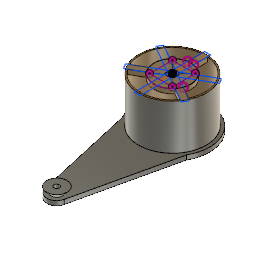
tulppajakiristinhuuli v2 (Autodesk Fusion 360 design; units mm, degrees)
Autodesk Fusion 360 part; units mm, degrees
note: some values were not read from the file. Set by a fixed rule: which sketch regions a step uses.
sketch "Sketch1" plane through (0, 0, 0) normal (0, 0, 1) x (1, 0, 0)
  circle A0 centre (0, 0) radius 48.5
  circle A1 centre (0, 0) radius 44.15
  circle A2 centre (0, 0) radius 42.15
  circle A3 centre (0, 0) radius 24
  line L0 (-4, 0) -> (4, 0)
  line L1 (4, 0) -> (4, 46)
  line L2 (4, 46) -> (-4, 46)
  line L3 (-4, 46) -> (-4, 0)
  line L4 (-2, 3.4641) -> (-41.8372, -19.5359)
  line L5 (-41.8372, -19.5359) -> (-37.8372, -26.4641)
  line L6 (-37.8372, -26.4641) -> (2, -3.4641)
  line L7 (2, -3.4641) -> (-2, 3.4641)
  line L8 (-2, -3.4641) -> (37.8372, -26.4641)
  line L9 (37.8372, -26.4641) -> (41.8372, -19.5359)
  line L10 (41.8372, -19.5359) -> (2, 3.4641)
  line L11 (2, 3.4641) -> (-2, -3.4641)
  circle A4 centre (0, 0) radius 6
  line L12 (15, 15) -> (-15, 15)
  line L13 (-15, 15) -> (-15, -15)
  line L14 (-15, -15) -> (15, -15)
  line L15 (15, -15) -> (15, 15)
  line L16 (15, 15) -> (-15, -15) construction
  line L17 (-15, 15) -> (15, -15) construction
  dimension "d1" = 97
  dimension "d2" = 88.3
  dimension "d3" = 84.3
  dimension "d4" = 48
  dimension "d6" = 360
  dimension "d7" = 12
  dimension "d12" = 30
  dimension "d13" = 30
  constraint coincident A0.centre A1.centre
  constraint concentric A1 A2
  constraint horizontal L0
  constraint vertical L1
  constraint horizontal L2
  constraint vertical L3
  constraint concentric A1 A4
  constraint perpendicular L12 L13
  constraint parallel L12 L14
  constraint parallel L13 L15
  constraint horizontal L12
  constraint coincident L16 A0.centre
  constraint coincident L17 A0.centre
  measures "d1" diameter of A0
  measures "d2" diameter of A1
  measures "d3" diameter of A2
  measures "d4" diameter of A3
  measures "d7" diameter of A4
  measures "d12" distance of L13.end L14.end
  measures "d13" distance of L12.end L13.end
extrude "Extrude1" add sketch "Sketch1" along normal blind 6 contours A0 | A1 L1 L2 L3 | A1 L8 L9 L10 | A2 A3 L1 L3 | A2 A3 L8 L10 | A1 L4 L5 L6 | A2 A3 L4 L6 | L1 L10 A4 L12 L15 | L1 L3 A4 L12 | L8 L10 A4 L15 | L3 L4 A4 L12 L13 | L6 L8 A4 L13 L14 L15 | L4 L6 A4 L13 makes body 1 at (48.4397, -2.4175, 4) makes body 2 at (-3.113, 29.8622, 0) makes body 3 at (-0.1495, -11.9944, 0) makes body 4 at (-27.4179, -12.2352, 0) makes body 5 at (27.4179, -12.2352, 0)
extrude "Extrude6" add sketch "Sketch1" along normal blind 6 contours A3 L1 L3 L12 | A3 L1 L10 L12 L15 | A3 L8 L10 L15 | A3 L3 L4 L12 L13 | A3 L6 L8 L13 L14 L15 | A3 L4 L6 L13 bodies 3 4 2 5
sketch "Sketch2" plane through (0, 0, 0) normal (0, 0, 1) x (1, 0, 0)
extrude "Extrude2" add sketch "Sketch1" along normal blind 65 contours A1 A2 L1 L10 | A1 A2 L1 L3 | A1 A2 L8 L10 | A1 A2 L3 L4 | A1 A2 L6 L8 | A1 A2 L4 L6 bodies 1 3
sketch "Sketch4" plane through (0, 0, 65) normal (0, 0, 1) x (-1, 0, 0)
  circle A0 centre (0, 0) radius 42.15
  circle A1 centre (0, 0) radius 44.15
  line L0 (-3.9193, -45.9529) -> (3.9193, -45.9529)
  line L1 (3.9193, -45.9529) -> (3.9193, 45.9529)
  line L2 (3.9193, 45.9529) -> (-3.9193, 45.9529)
  line L3 (-3.9193, 45.9529) -> (-3.9193, -45.9529)
  line L4 (-3.9193, -45.9529) -> (3.9193, 45.9529) construction
  line L5 (3.9193, -45.9529) -> (-3.9193, 45.9529) construction
  line L6 (41.7561, 19.5823) -> (37.8368, 26.3707)
  line L7 (-37.8368, -26.3707) -> (41.7561, 19.5823)
  line L8 (37.8368, 26.3707) -> (-41.7561, -19.5823)
  line L9 (-41.7561, -19.5823) -> (-37.8368, -26.3707)
  line L10 (-37.8368, 26.3707) -> (-41.7561, 19.5823)
  line L11 (41.7561, -19.5823) -> (-37.8368, 26.3707)
  line L12 (-41.7561, 19.5823) -> (37.8368, -26.3707)
  line L13 (37.8368, -26.3707) -> (41.7561, -19.5823)
  circle A2 centre (0, 0) radius 6
  circle A3 centre (0, 0) radius 24
  line L14 (-15, 15) -> (15, 15)
  line L15 (15, 15) -> (15, -15)
  line L16 (15, -15) -> (-15, -15)
  line L17 (-15, -15) -> (-15, 15)
  line L18 (-15, 15) -> (15, -15) construction
  line L19 (15, 15) -> (-15, -15) construction
  dimension "d20" = 360
  dimension "d21" = 12
  dimension "d22" = 48
  dimension "d25" = 30
  dimension "d26" = 30
  constraint perpendicular L0 L1
  constraint parallel L0 L2
  constraint parallel L1 L3
  constraint horizontal L0
  constraint coincident L4 A0.centre
  constraint coincident L5 A0.centre
  constraint coincident A0.centre A1.centre
  constraint concentric A0 A2
  constraint concentric A0 A3
  constraint perpendicular L14 L15
  constraint parallel L14 L16
  constraint parallel L15 L17
  constraint horizontal L14
  constraint coincident L18 A0.centre
  constraint coincident L19 A0.centre
  measures "d21" diameter of A2
  measures "d22" diameter of A3
  measures "d25" distance of L15.end L16.end
  measures "d26" distance of L14.end L15.end
extrude "Extrude4" add sketch "Sketch4" against normal blind 6 contours A0 L7 L8 A3 | L7 L11 A3 L15 | L7 L8 A3 L15 | L11 L12 A3 L15 | L1 L8 A3 L14 L15 | A0 L1 L3 A3 | L1 L12 A3 L15 L16 | L1 L3 A3 L14 | L1 L3 A3 L16 | A0 L11 L12 A3 | L3 L11 A3 L14 L17 | L3 L7 A3 L16 L17 | L11 L12 A3 L17 | L7 L8 A3 L17 | L8 L12 A3 L17 picked at (24.3429, 17.5763) picked at (3.0501, -29.8698) picked at (-27.393, 12.2934) bodies 1
sketch "Sketch5" plane through (0, 0, 65) normal (0, 0, 1) x (-1, 0, 0)
  arc A0 (3.9193, -41.9674) -> (38.3045, 17.5895) centre (0, 0) ccw
  line L0 (3.9193, -41.9674) -> (3.9193, -23.6778)
  arc A1 (3.9193, -23.6778) -> (22.4652, 8.4447) centre (0, 0) ccw
  line L1 (22.4652, 8.4447) -> (38.3045, 17.5895)
  line L2 (34.3852, 24.3779) -> (18.5459, 15.2331)
  line L3 (-18.5459, 15.2331) -> (-34.3852, 24.3779)
  arc A2 (34.3852, 24.3779) -> (-34.3852, 24.3779) centre (0, 0) ccw
  line L4 (-38.3045, 17.5895) -> (-22.4652, 8.4447)
  arc A3 (-22.4652, 8.4447) -> (-3.9193, -23.6778) centre (0, 0) ccw
  line L5 (-3.9193, -23.6778) -> (-3.9193, -41.9674)
  arc A4 (-38.3045, 17.5895) -> (-3.9193, -41.9674) centre (0, 0) ccw
  circle A5 centre (0, 0) radius 44.15
  arc A6 (18.5459, 15.2331) -> (-18.5459, 15.2331) centre (0, 0) ccw
  line L6 (15, -15) -> (-15, -15)
  line L7 (-15, -15) -> (-15, 15)
  line L8 (-15, 15) -> (15, 15)
  line L9 (15, 15) -> (15, -15)
extrude "Extrude5" add sketch "Sketch4" against normal blind 3 contours L7 L11 L15 | L1 L7 L8 L11 A2 L15 | L1 L7 L11 L12 A2 L15 | L1 L8 L14 L15 | L7 L11 A2 | L1 L12 L15 L16 | L1 L3 L8 L11 A2 L14 | L1 L8 A2 | L1 L3 L7 L12 A2 L16 | L1 L12 A2 | L3 L11 L14 L17 | L3 L7 L16 L17 | L3 L8 L11 L12 A2 L17 | L3 L11 A2 | L3 L7 L8 L12 A2 L17 | L3 L7 A2 | L8 L12 L17 | L8 L12 A2 bodies 1
extrude "Extrude7" add sketch "Sketch4" against normal blind 6 contours L7 L11 L15 | L1 L7 L8 L11 A2 L15 | L1 L7 L11 L12 A2 L15 | L1 L8 L14 L15 | L7 L11 A2 | L1 L12 L15 L16 | L1 L3 L8 L11 A2 L14 | L1 L8 A2 | L1 L3 L7 L12 A2 L16 | L1 L12 A2 | L3 L11 L14 L17 | L3 L7 L16 L17 | L3 L8 L11 L12 A2 L17 | L3 L11 A2 | L3 L7 L8 L12 A2 L17 | L3 L7 A2 | L8 L12 L17 | L8 L12 A2 bodies 1
sketch "Sketch8" plane through (0, 0, 0) normal (0, 0, 1) x (1, 0, 0)
sketch "Sketch9" plane through (0, 0, 0) normal (0, 0, 1) x (1, 0, 0)
  line L0 (10, 10) -> (-10, 10)
  line L1 (-10, 10) -> (-10, -10)
  line L2 (-10, -10) -> (10, -10)
  line L3 (10, -10) -> (10, 10)
  line L4 (10, 10) -> (-10, -10) construction
  line L5 (-10, 10) -> (10, -10) construction
  dimension "d33" = 20
  constraint perpendicular L0 L1
  constraint parallel L0 L2
  constraint parallel L1 L3
  constraint horizontal L0
  constraint coincident L4 origin
  constraint coincident L5 origin
  measures "d33" distance of L1.end L2.end
sketch "Sketch10" plane through (0, 0, 0) normal (0, 0, 1) x (1, 0, 0)
sketch "Sketch13" plane through (0, 0, 0) normal (0, 0, -1) x (1, 0, 0)
  arc A0 (4, -41.9598) -> (38.3382, 17.5158) centre (0, 0) ccw
  line L0 (4, -41.9598) -> (4, -23.6643)
  arc A1 (4, -23.6643) -> (22.4939, 8.3681) centre (0, 0) ccw
  line L1 (22.4939, 8.3681) -> (38.3382, 17.5158)
  arc A2 (-38.3382, 17.5158) -> (-4, -41.9598) centre (0, 0) ccw
  line L2 (-38.3382, 17.5158) -> (-22.4939, 8.3681)
  arc A3 (-22.4939, 8.3681) -> (-4, -23.6643) centre (0, 0) ccw
  line L3 (-4, -23.6643) -> (-4, -41.9598)
  circle A4 centre (0, 0) radius 6
  line L4 (34.3382, 24.444) -> (18.4939, 15.2963)
  arc A5 (18.4939, 15.2963) -> (-18.4939, 15.2963) centre (0, 0) ccw
  line L5 (-18.4939, 15.2963) -> (-34.3382, 24.444)
  arc A6 (34.3382, 24.444) -> (-34.3382, 24.444) centre (0, 0) ccw
  circle A7 centre (0, 0) radius 48.5
sketch "Sketch14" plane through (0, 0, 0) normal (0, 0, -1) x (1, 0, 0)
  line L0 (0, 0) -> (0, 210)
  line L1 (0, 210) -> (47.0531, 2.6393)
  line L2 (47.0531, 2.6393) -> (-47.1343, 2.6393)
  line L3 (-47.1343, 2.6393) -> (0, 210)
  dimension "d54" = 210
  constraint coincident L0.start origin
  constraint vertical L0
  constraint perpendicular L0 L2
  measures "d54" distance of L0.start L0.end
extrude "Extrude8" add sketch "Sketch14" against normal blind 6 bodies 1
fillet "Fillet1" radius 13 1 edges at (0, -210, 3) on bodies 1
extrude "Extrude9" cut sketch "Sketch9" sketch "Sketch1" along normal blind 2 of sketch 2 contours L1 L10 A4 L12 L15 | L1 L3 A4 L12 | L8 L10 A4 L15 | L3 L4 A4 L12 L13 | L6 L8 A4 L13 L14 L15 | L4 L6 A4 L13 bodies 1
extrude "Extrude10" cut sketch "Sketch13" against normal blind 11 contours A4 bodies 1
sketch "Sketch15" plane through (0, 0, 0) normal (0, 0, -1) x (1, 0, 0)
  line L0 (-15, 15) -> (15, 15)
  line L1 (15, 15) -> (15, -15)
  line L2 (15, -15) -> (-15, -15)
  line L3 (-15, -15) -> (-15, 15)
  arc A0 (12.6668, 154.1781) -> (-12.6876, 154.1828) centre (-0.0109, 151.3013) ccw
  line L4 (-12.6876, 154.1828) -> (-42.3691, 23.6032)
  arc A1 (-42.3691, 23.6032) -> (42.2464, 23.8222) centre (0, 0) ccw
  line L5 (42.2464, 23.8222) -> (12.6668, 154.1781)
  arc A2 (-23.8544, 2.6393) -> (-4, -23.6643) centre (0, 0) ccw
  line L6 (-4, -23.6643) -> (-4, -41.9598)
  arc A3 (-42.0673, 2.6393) -> (-4, -41.9598) centre (0, 0) ccw
  line L7 (-42.0673, 2.6393) -> (-23.8544, 2.6393)
  line L8 (23.8544, 2.6393) -> (42.0673, 2.6393)
  arc A4 (4, -41.9598) -> (42.0673, 2.6393) centre (0, 0) ccw
  line L9 (4, -41.9598) -> (4, -23.6643)
  arc A5 (4, -23.6643) -> (23.8544, 2.6393) centre (0, 0) ccw
sketch "Sketch16" plane through (0, 0, 6) normal (0, 0, 1) x (-1, 0, 0)
  arc A0 (12.6876, 154.1828) -> (-12.6668, 154.1781) centre (0.0109, 151.3013) ccw
  line L0 (-12.6668, 154.1781) -> (-42.2464, 23.8222)
  arc A1 (-42.2464, 23.8222) -> (42.3691, 23.6032) centre (0, 0) ccw
  line L1 (42.3691, 23.6032) -> (12.6876, 154.1828)
  circle A2 centre (0, 0) radius 44.15
  circle A3 centre (0.0109, 151.3013) radius 7.5884
extrude "Extrude11" add sketch "Sketch16" along normal blind 7 draft 40 contours A3 bodies 1
hole "Hole7" at (-0.0109, -151.3013, 0) direction (0, 0, 1) diameter 7.05 depth 22 tip angle 180 bodies 1
